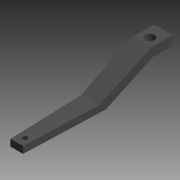
# Autodesk Inventor part: shift_lever
Saved by Autodesk Inventor 2015 (Build 190159000, 159)
## iProperties
Created: 2015-10-08
Part Number: shift_lever
Material: Generic
Document SubType Name: Modeling
Designer: c3132704
Appearance: Generic
Author: c3132704
Autodesk Inventor part; units mm, degrees
ref_plane "YZ Plane" through (0, 0, 0) normal (1, 0, 0) x (0, 1, 0)
ref_plane "XZ Plane" through (0, 0, 0) normal (0, 1, 0) x (-1, 0, 0)
ref_plane "XY Plane" through (0, 0, 0) normal (0, 0, 1) x (1, 0, 0)
sketch "Sketch1" plane through (0, 0, 0) normal (1, 0, 0) x (0, 1, 0)
  line L0 (-13.5824, 59.2417) -> (-13.5824, -35.4929)
  line L1 (-13.5824, -35.4929) -> (12.4176, -91.2501)
  line L2 (12.4176, -91.2501) -> (12.4176, -114.7505)
  line L3 (12.4176, -114.7505) -> (23.4176, -114.7505)
  line L4 (23.4176, -114.7505) -> (23.4176, -89.7505)
  line L5 (23.4176, -89.7505) -> (-5.5824, -27.5598)
  line L6 (-5.5824, -27.5598) -> (-5.5824, 59.2417)
  line L7 (-5.5824, 59.2417) -> (-13.5824, 59.2417)
  point P0 (0, 0)
  dimension "d0" = 8
  dimension "d1" = 173.9922
  dimension "d2" = 25
  dimension "d3" = 37
  dimension "d4" = 11
  dimension "d5" = 155
  constraints: 16 end point, 3 parallel, 3 perpendicular, 1 vertical
  measures "d0" distance between parallel lines of L0 L6
  measures "d1" distance between parallel lines of L3 L7
  measures "d2" distance of L3.end L4.end
  measures "d3" distance between parallel lines of L0 L4
  measures "d4" distance of L2.end L3.end
  measures "d5" angle of L6 L5
extrude "Extrusion1" add sketch "Sketch1" along normal blind 22
chamfer "Chamfer1" distance 100 distance2 3.5 1 edges at (22, -9.5824, 59.2417) measured on face at (22, -9.5824, 58.7417)
chamfer "Chamfer2" distance 100 distance2 3.5 1 edges at (0, -9.5824, 59.2417) measured on face at (0, -9.5824, 58.7417)
hole "Hole1" at (11, -5.5824, 50.2417) direction (0, -1, 0) diameter 6 end through all
hole "Hole2" at (11, 23.4176, -98.7505) direction (0, -1, 0) diameter 11 end through all
body "Solid1"
